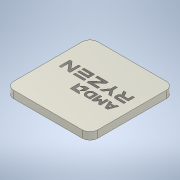
# Autodesk Inventor part: Ryzen IHS
Saved by Autodesk Inventor 2020 (Build 240168000, 168)
## iProperties
Created: 2020-11-28
Part Number: Ryzen IHS
Material: Kupfer
Document SubType Name: Modeling
Designer: david
Density: 8.94 g/cm^3
Appearance: Nickel
Author: david
Autodesk Inventor part; units mm, degrees
ref_plane "YZ Plane" through (0, 0, 0) normal (1, 0, 0) x (0, 1, 0)
ref_plane "XZ Plane" through (0, 0, 0) normal (0, 1, 0) x (-1, 0, 0)
ref_plane "XY Plane" through (0, 0, 0) normal (0, 0, 1) x (1, 0, 0)
sketch "Skizze1" plane through (0, 0, 0) normal (0, 1, 0) x (-1, 0, 0)
  line L0 (-18.75, 18.75) -> (18.75, 18.75)
  line L1 (18.75, 18.75) -> (18.75, -18.75)
  line L2 (18.75, -18.75) -> (-18.75, -18.75)
  line L3 (-18.75, -18.75) -> (-18.75, 18.75)
  line L4 (-18.75, 18.75) -> (18.75, -18.75) construction
  line L5 (18.75, 18.75) -> (-18.75, -18.75) construction
  point P0 (0, 0)
  dimension "d0" = 37.5
  dimension "d1" = 37.5
  constraints: 12 end point, 2 midpoint, 2 parallel, 1 horizontal, 1 perpendicular
  measures "d0" distance of L1.end L2.end
  measures "d1" distance of L0.end L1.end
extrude "Extrusion1" add sketch "Skizze1" against normal blind 3.25
fillet "Rundung1" radius 3.5 4 edges at (18.75, -1.625, 18.75) (-18.75, -1.625, 18.75) (18.75, -1.625, -18.75) (-18.75, -1.625, -18.75)
sketch "Skizze2" plane through (0, -3.25, 0) normal (0, -1, 0) x (1, 0, 0)
  arc A0 (-18.75, -15.25) -> (-15.25, -18.75) centre (-15.25, -15.25) ccw projected
  line L0 (-15.25, -18.75) -> (15.25, -18.75) projected
  arc A1 (15.25, -18.75) -> (18.75, -15.25) centre (15.25, -15.25) ccw projected
  line L1 (18.75, -15.25) -> (18.75, 15.25) projected
  arc A2 (18.75, 15.25) -> (15.25, 18.75) centre (15.25, 15.25) ccw projected
  line L2 (15.25, 18.75) -> (-15.25, 18.75) projected
  arc A3 (-15.25, 18.75) -> (-18.75, 15.25) centre (-15.25, 15.25) ccw projected
  line L3 (-18.75, 15.25) -> (-18.75, -15.25) projected
  line L4 (13.75, -15.75) -> (-13.75, -15.75)
  line L5 (-15.75, -13.75) -> (-15.75, 13.75)
  line L6 (-13.75, 15.75) -> (13.75, 15.75)
  line L7 (15.75, 13.75) -> (15.75, -13.75)
  arc A4 (13.75, -15.75) -> (15.75, -13.75) centre (13.75, -13.75) ccw
  arc A5 (-15.75, -13.75) -> (-13.75, -15.75) centre (-13.75, -13.75) ccw
  arc A6 (-13.75, 15.75) -> (-15.75, 13.75) centre (-13.75, 13.75) ccw
  arc A7 (15.75, 13.75) -> (13.75, 15.75) centre (13.75, 13.75) ccw
  point P0 (0, 0)
  dimension "d5" = 3
  dimension "d317" = 2
  dimension "d318" = 3
  dimension "d319" = 3
  constraints: 8 end point, 8 point on circle, 8 tangent, 4 centre point, 3 equal radius, 2 perpendicular, 1 horizontal, 1 vertical
  measures "d5" distance between parallel lines of L0 L4
  measures "d317" radius of A4
  measures "d318" distance between parallel lines of L3 L5
  measures "d319" distance between parallel lines of L1 L7
extrude "Extrusion2" cut sketch "Skizze2" against normal blind 0.8 contours L4 A5 L5 A6 L6 A7 L7 A4
sketch "Skizze3" plane through (0, 0, 0) normal (0, 1, 0) x (1, 0, 0)
  line L0 (-26.25, 0) -> (26.25, 0) construction
  line L1 (0, 26.25) -> (0, -26.25) construction
  line L2 (18.75, -12.5) -> (-18.75, -12.5) construction
  line L3 (-18.75, -12.5) -> (-18.75, 12.5) construction
  line L4 (-18.75, 12.5) -> (18.75, 12.5) construction
  line L5 (18.75, 12.5) -> (18.75, -12.5) construction
  line L6 (-18.75, 15.25) -> (-18.75, -15.25) projected
  line L7 (18.75, -15.25) -> (18.75, 15.25) projected
  line L8 (14.4327, -1.4997) -> (13.4446, -1.4997)
  line L9 (13.4446, -1.4997) -> (13.1723, -2.2216)
  line L10 (13.1723, -2.2216) -> (11.539, -2.2269)
  line L11 (11.539, -2.2269) -> (11.2323, -1.4997)
  line L12 (11.2323, -1.4997) -> (10.2223, -1.4997)
  line L13 (10.2223, -1.4997) -> (11.8654, -5.1845)
  line L14 (11.8654, -5.1845) -> (12.9419, -5.1845)
  line L15 (12.9419, -5.1845) -> (14.4327, -1.4997)
  line L16 (12.9231, -2.8778) -> (12.3965, -4.2783)
  line L17 (12.3965, -4.2783) -> (11.8135, -2.8778)
  line L18 (11.8135, -2.8778) -> (12.9231, -2.8778)
  line L19 (9.8245, -1.5018) -> (9.8245, -5.1845)
  line L20 (9.8245, -5.1845) -> (9.0017, -5.1845)
  line L21 (9.0017, -5.1845) -> (7.8384, -3.8416)
  line L22 (7.8384, -3.8416) -> (6.6605, -5.1845)
  line L23 (6.6605, -5.1845) -> (5.8519, -5.1845)
  line L24 (5.8519, -5.1845) -> (5.8519, -1.5018)
  line L25 (5.8519, -1.5018) -> (6.774, -1.5018)
  line L26 (6.774, -1.5018) -> (6.774, -3.7836)
  line L27 (6.774, -3.7836) -> (7.7567, -2.6427)
  line L28 (7.7567, -2.6427) -> (7.9104, -2.6427)
  line L29 (7.9104, -2.6427) -> (8.8888, -3.7836)
  line L30 (8.8888, -3.7836) -> (8.8888, -1.5018)
  line L31 (8.8888, -1.5018) -> (9.8245, -1.5018)
  line L32 (5.1627, -5.1845) -> (3.3425, -5.1845)
  line L33 (3.3425, -5.1845) -> (3.3227, -5.1845)
  line L34 (1.4935, -3.3726) -> (1.4935, -3.3726)
  line L35 (5.1627, -1.4997) -> (3.3227, -1.4997)
  line L36 (1.4827, -3.3798) -> (1.4827, -3.2557)
  ellipse E0 centre (3.3227, -3.3798) end of major axis (3.3227, -5.1845) minor radius 1.84 (1.4838, -3.3169) -> (3.3227, -5.1845) ccw
  ellipse E1 centre (3.3227, -3.2557) end of major axis (3.3227, -5.0116) minor radius 1.84 (3.3227, -1.4997) -> (1.4838, -3.3169) ccw
  line L37 (5.1627, -5.1845) -> (5.1627, -1.4997)
  line L38 (4.2279, -4.4992) -> (4.2279, -2.1929)
  line L39 (4.2279, -2.1929) -> (3.4947, -2.1929)
  arc A0 (3.4947, -2.1929) -> (2.4503, -3.2373) centre (3.4947, -3.2373) ccw
  line L40 (2.4503, -3.2373) -> (2.4503, -3.4636)
  arc A1 (2.4503, -3.4636) -> (3.4859, -4.4992) centre (3.4859, -3.4636) ccw
  line L41 (3.4859, -4.4992) -> (4.2279, -4.4992)
  line L42 (0.8602, -1.2135) -> (0.8602, -2.8933)
  line L43 (0.8602, -2.8933) -> (-0.3342, -4.09)
  line L44 (-0.3342, -4.09) -> (-0.3342, -2.4126)
  line L45 (-0.3342, -2.4126) -> (-2.0149, -2.4126)
  line L46 (-2.0149, -2.4126) -> (-0.8181, -1.2135)
  line L47 (-0.8181, -1.2135) -> (0.8602, -1.2135)
  line L48 (0.823, -5.474) -> (-3.3997, -5.474)
  line L49 (-3.3997, -5.474) -> (-3.3997, -1.2507)
  line L50 (-3.3997, -1.2507) -> (-3.3785, -1.2507)
  line L51 (-3.3785, -1.2507) -> (-2.2269, -2.4042)
  line L52 (-2.2269, -2.4042) -> (-2.2269, -4.2998)
  line L53 (-2.2269, -4.2998) -> (-0.328, -4.2998)
  line L54 (-0.328, -4.2998) -> (0.823, -5.4569)
  line L55 (0.823, -5.4569) -> (0.823, -5.474)
  line L56 (14.4279, 0.6783) -> (14.4279, 1.6389)
  line L57 (14.4279, 1.6389) -> (10.665, 1.6389)
  arc A2 (10.6027, 1.7012) -> (10.665, 1.6389) centre (10.665, 1.7012) ccw
  line L58 (10.6027, 1.7012) -> (10.603, 2.5347)
  arc A3 (10.658, 2.5896) -> (10.603, 2.5347) centre (10.6579, 2.5346) ccw
  line L59 (10.658, 2.5896) -> (14.4279, 2.5915)
  line L60 (14.4279, 2.5915) -> (14.4279, 5.4762)
  line L61 (14.4279, 5.4762) -> (13.4636, 5.4762)
  line L62 (13.4636, 5.4762) -> (13.4629, 3.5488)
  line L63 (13.4629, 3.5488) -> (11.7096, 3.5495)
  line L64 (11.7096, 3.5495) -> (10.6041, 5.4762)
  line L65 (10.6041, 5.4762) -> (9.4784, 5.4762)
  line L66 (9.4784, 5.4762) -> (10.5768, 3.5617)
  arc A4 (10.5768, 3.5617) -> (9.6302, 2.5811) centre (10.6114, 2.5811) ccw
  line L67 (9.6302, 2.5811) -> (9.6302, 1.6)
  arc A5 (9.6302, 1.6) -> (10.5518, 0.6783) centre (10.5518, 1.6) ccw
  line L68 (10.5518, 0.6783) -> (14.4279, 0.6783)
  line L69 (8.8236, 0.6783) -> (7.6223, 0.6783)
  line L70 (7.6223, 0.6783) -> (6.2562, 2.5641)
  line L71 (6.2562, 2.5641) -> (4.8968, 0.6783)
  line L72 (4.8968, 0.6783) -> (3.6896, 0.6759)
  line L73 (3.6896, 0.6759) -> (5.773, 3.5418)
  line L74 (5.773, 3.5418) -> (5.773, 5.4762)
  line L75 (5.773, 5.4762) -> (6.7507, 5.4762)
  line L76 (6.7507, 5.4762) -> (6.7507, 3.5514)
  line L77 (6.7507, 3.5514) -> (8.8236, 0.6783)
  line L78 (2.734, 0.674) -> (-2.0615, 0.674)
  line L79 (-2.0615, 0.674) -> (-2.0615, 1.6467)
  line L80 (-2.0615, 1.6467) -> (1.248, 4.4985)
  line L81 (1.248, 4.4985) -> (-2.0615, 4.4985)
  line L82 (-2.0615, 4.4985) -> (-2.0615, 5.4762)
  line L83 (-2.0615, 5.4762) -> (2.7344, 5.4744)
  line L84 (2.7344, 5.4744) -> (2.734, 4.4903)
  line L85 (2.734, 4.4903) -> (-0.5827, 1.6379)
  line L86 (-0.5827, 1.6379) -> (2.734, 1.6366)
  line L87 (2.734, 1.6366) -> (2.734, 0.674)
  line L88 (-3.3891, 0.6783) -> (-8.1877, 0.6783)
  line L89 (-8.1877, 0.6783) -> (-8.1877, 1.6366)
  line L90 (-8.1877, 1.6366) -> (-3.3891, 1.6366)
  line L91 (-3.3891, 1.6366) -> (-3.3891, 0.6783)
  line L92 (-3.3891, 2.5896) -> (-8.1877, 2.5896)
  line L93 (-8.1877, 5.4744) -> (-3.3891, 5.4744)
  line L94 (-3.3891, 5.4744) -> (-3.3891, 2.5896)
  line L95 (-4.3624, 3.5617) -> (-8.1877, 3.5617)
  line L96 (-8.1877, 4.5002) -> (-4.3624, 4.5002)
  line L97 (-4.3624, 4.5002) -> (-4.3624, 3.5617)
  line L98 (-8.1877, 2.5896) -> (-8.1877, 3.5617)
  line L99 (-8.1877, 4.5002) -> (-8.1877, 5.4744)
  line L100 (-9.6256, 5.4735) -> (-9.6256, 0.6759)
  line L101 (-9.6256, 0.6759) -> (-10.6094, 0.6759)
  line L102 (-10.6094, 0.6759) -> (-13.4614, 3.9922)
  line L103 (-13.4614, 3.9922) -> (-13.4643, 0.6759)
  line L104 (-13.4643, 0.6759) -> (-14.4237, 0.6759)
  line L105 (-14.4237, 0.6759) -> (-14.4237, 5.4744)
  line L106 (-14.4237, 5.4744) -> (-13.4516, 5.4744)
  line L107 (-13.4516, 5.4744) -> (-10.6004, 2.1628)
  line L108 (-10.6004, 2.1628) -> (-10.5975, 5.4744)
  line L109 (-10.5975, 5.4744) -> (-9.6256, 5.4735)
  point P0 (0, 0)
  dimension "d256" = 4.3173
  dimension "d257" = 1.4997
  dimension "d258" = 3.6848
  constraints: 205 end point, 28 perpendicular, 23 point on line, 19 parallel, 15 horizontal, 12 point on circle, 10 vertical, 9 tangent, 6 centre point, 11 other
  measures "d256" distance from line of L7 L8.start
  measures "d257" distance between parallel lines of L0 L8
  measures "d258" distance between parallel lines of L12 L14
emboss "Prägen1" sketch "Skizze3" operation cut depth 0.01 direction (0, -1, 0)
